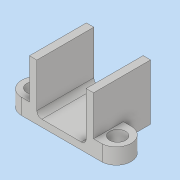
# Autodesk Inventor part: N20电机座
Saved by Autodesk Inventor 2019 (Build 230136000, 136)
## iProperties
Created: 2020-11-03
Part Number: N20电机座
Material: Generic
Document SubType Name: Modeling
Designer: Wang Hua
Density: 1 g/cm^3
Appearance: Default
Author: Wang Hua
Autodesk Inventor part; units mm, degrees
ref_plane "YZ Plane" through (0, 0, 0) normal (1, 0, 0) x (0, 1, 0)
ref_plane "XZ Plane" through (0, 0, 0) normal (0, 1, 0) x (-1, 0, 0)
sketch "草图1" plane through (0, 0, 0) normal (0, 0, 1) x (1, 0, 0)
  line L0 (-6.475, -5.625) -> (6.475, -5.625)
  line L1 (6.475, -5.625) -> (6.475, 5.625)
  line L2 (6.475, 5.625) -> (-6.475, 5.625)
  line L3 (-6.475, 5.625) -> (-6.475, -5.625)
  line L4 (-6.475, -5.625) -> (6.475, 5.625) construction
  line L5 (6.475, -5.625) -> (-6.475, 5.625) construction
  line L6 (4.975, -4.225) -> (-4.975, -4.225)
  line L7 (-4.975, -4.225) -> (-4.975, 5.625)
  line L8 (-4.975, 5.625) -> (4.975, 5.625)
  line L9 (4.975, 5.625) -> (4.975, -4.225)
  line L10 (4.975, -4.225) -> (-4.975, 5.625) construction
  line L11 (-4.975, -4.225) -> (4.975, 5.625) construction
  line L12 (0, -7.875) -> (0, 7.875) projected
  point P0 (0, 0)
  point P1 (0, 0.7)
  point P2 (0, 0.7)
  dimension "d0" = 11.25
  dimension "d1" = 9.85
  dimension "d2" = 9.95
  dimension "d3" = 1.5
  constraints: 24 end point, 5 midpoint, 4 parallel, 2 horizontal, 2 perpendicular, 1 collinear, 1 point on line
  measures "d0" distance of L2.end L0.start
  measures "d1" distance of L6.end L7.end
  measures "d2" distance between parallel lines of L9 L7
  measures "d3" distance between parallel lines of L3 L7
extrude "拉伸1" add sketch "草图1" along normal blind 11.5 contours L3 L2 L7 L6 L12 L0 | L12 L6 L9 L2 L1 L0
sketch "草图2" plane through (-6.475, -5.625, 0) normal (0, -1, 0) x (1, 0, 0)
  line L0 (0, 0) -> (12.95, 0) projected
  line L1 (12.95, 0) -> (12.95, 11.5) projected
  line L2 (0, 11.5) -> (12.95, 11.5) projected
  line L3 (0, 0) -> (0, 11.5) projected
  line L4 (0, 11.5) -> (12.95, 11.5) construction
  line L5 (6.475, 11.5) -> (6.475, 0) construction
  line L6 (12.95, 11.5) -> (11.45, 11.5) construction
  line L7 (12.95, 11.5) -> (14.65, 11.5)
  line L8 (12.95, 0) -> (12.95, 11.5) construction
  line L9 (12.95, 5.505) -> (14.65, 5.505)
  arc A0 (14.65, 5.505) -> (14.65, 11.5) centre (14.5281, 8.5025) ccw
  line L10 (0, 11.5) -> (-1.7, 11.5)
  line L11 (0, 5.505) -> (-1.7, 5.505)
  arc A1 (-1.7, 11.5) -> (-1.7, 5.505) centre (-1.5781, 8.5025) ccw
  point P0 (14.85, 8.55)
  point P1 (-1.9, 8.55)
  dimension "d6" = 1.7
  dimension "d7" = 3
  dimension "d8" = 1.9
  dimension "d9" = 2.95
  constraints: 10 end point, 5 symmetric about line, 4 point on circle, 2 centre point, 2 point on line, 1 horizontal, 1 midpoint, 1 parallel, 1 perpendicular, 1 vertical, 1 other
  measures "d6" distance of L1.end L7.end
  measures "d7" radius of A0
  measures "d8" distance from line of L1 point (14.85, 8.55)
  measures "d9" distance from line of L7 point (14.85, 8.55)
extrude "拉伸2" add sketch "草图2" against normal blind 3.2 contours L1 L7 A0 L9
ref_plane "工作平面1" through (0, -5.625, 0) normal (1, 0, 0) x (0, 0, -1)
mirror "镜像1" about plane through (0, -5.625, 0) normal (1, 0, 0) of "拉伸2"
hole "孔1" at (8.375, -5.625, 8.55) at (-8.375, -5.625, 8.55) direction (0, 1, 0) diameter 3.2 end through all
fillet "圆角1" radius 1 2 edges at (4.975, -4.225, 5.75) (-4.975, -4.225, 5.75)
